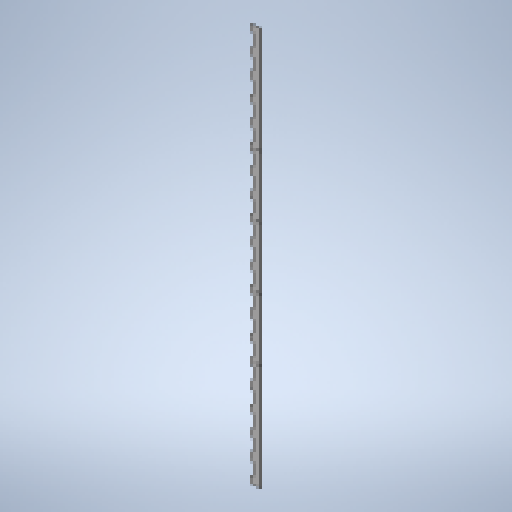
# Autodesk Inventor part: BSH 046 stringer 61
Saved by Autodesk Inventor 2025 (Build 290162010, 162A)
## iProperties
Created: 2024-07-23
Part Number: BSH 046 stringer 61
Material: 09g2s
Document SubType Name: Sheet Metal
Designer: pokla
Mass: 3171.2 g
Surface Area: 2845.67 cm^2
Volume: 403.975 cm^3
Density: 7.85 g/cm^3
Flat Pattern Width: 7.02891 cm
Flat Pattern Length: 289.7 cm
Flat Pattern Area: 2036.27 cm^2
Sheet Metal Rule: AISI304 3mm Die 32
Sheet Metal Width: 70,289 mm
Sheet Metal Length: 2897,000 mm
Sheet Metal Area: 203627,492 mm^2
Appearance: Default
Author: admin
Autodesk Inventor part; units mm, degrees
ref_plane "YZ Plane" through (0, 0, 0) normal (1, 0, 0) x (0, 1, 0)
ref_plane "XZ Plane" through (0, 0, 0) normal (0, 1, 0) x (-1, 0, 0)
ref_plane "XY Plane" through (0, 0, 0) normal (0, 0, 1) x (1, 0, 0)
sketch "Sketch6" plane through (0, 0, 0) normal (0, 1, 0) x (-1, 0, 0)
  line L0 (0, -1448.5) -> (-70.2891, -1448.5)
  line L1 (-70.2891, -1448.5) -> (-70.2891, 1448.5)
  line L2 (-70.2891, 1448.5) -> (0, 1448.5)
  line L3 (0, 1448.5) -> (0, -1448.5)
  point P0 (0, 0)
  point P1 (0, 0)
  dimension "d26" = 70.2891
  dimension "d27" = 2897
  measures "d26" distance of L1.end L2.end
  measures "d27" distance of L0.end L1.end
extrude "Plate4" add sketch "Sketch6" along normal blind 3
sketch "Sketch7" plane through (0, 0, 0) normal (0, -1, 0) x (1, 0, 0)
  line L0 (0, 1448.5) -> (70.2891, 1448.5) projected
  line L1 (0, -1448.5) -> (0, 1448.5) projected
  line L2 (70.2891, -1448.5) -> (0, -1448.5) projected
  line L3 (70.2891, 1448.5) -> (70.2891, -1448.5) projected
  line L4 (20, -30) -> (20, 30)
  arc A0 (0, -50) -> (20, -30) centre (0, -30) ccw
  arc A1 (20, 30) -> (0, 50) centre (0, 30) ccw
  point P0 (0, 0)
  point P1 (20, 0)
  point P2 (0, 0)
  dimension "d37" = 20
  dimension "d38" = 100
  constraints: 4 point on circle, 4 point on line, 2 centre point, 2 end point, 2 midpoint, 2 tangent, 1 horizontal alignment, 1 vertical
  measures "d37" distance between parallel lines of L1 L4
  measures "d38" distance of A1.end A0.start
extrude "Extrusion2" cut sketch "Sketch7" against normal through all contours A1 L4 A0 L1
pattern_linear "Rectangular Pattern2" count 19 spacing 150 along (0, 0, 1) of "Extrusion2" first direction both ways yes
sketch "Sketch8" plane through (0, 0, 0) normal (0, -1, 0) x (1, 0, 0)
  line L0 (70.2891, 1448.5) -> (70.2891, -1448.5) projected
  line L1 (0, -1277.1) -> (36.289, -1277.1)
  line L2 (36.289, -1277.1) -> (36.289, -1273.9)
  line L3 (36.289, -1273.9) -> (0, -1273.9)
  line L4 (0, -1273.9) -> (0, -1277.1)
  point P0 (0, 0)
  point P1 (0, -1275.5)
  point P2 (0, -1448.5)
  dimension "d57" = 3.2
  dimension "d58" = 36.289
  dimension "d59" = 173
  constraints: 8 end point, 2 parallel, 1 horizontal, 1 midpoint, 1 perpendicular, 1 vertical alignment
  measures "d57" distance between parallel lines of L3 L1
  measures "d58" distance of L2.end L3.end
  measures "d59" distance of point (0, -1448.5) point (0, -1275.5)
extrude "Extrusion4" cut sketch "Sketch8" against normal through all
pattern_linear "Rectangular Pattern3" count 5 spacing 450 along (0, 0, 1) of "Extrusion4"
equation "\"d26\" = Stringer3_deep"
equation "\"d28\" = Thickness"
equation "\"BendReliefWidth\" = Thickness"
equation "\"BendReliefDepth\" = 0.5 * Thickness"
equation "\"CornerReliefSize\" = 4 * Thickness"
equation "\"MinimumRemnant\" = 2 * Thickness"
equation "\"TransitionRadius\" = BendRadius"
equation "\"JacobiRadiusSize\" = BendRadius"
equation "\"GapSize\" = Thickness"
equation "\"Stringer3_deep\" = 70.28909"
equation "\"Thickness\" = 3"
equation "\"BendRadius\" = 5"
body "Solid2"
